Autodesk Inventor part; units mm, degrees
(part 2 of 9)
sketch "Sketch19" plane through (0, 0, 0) normal (1, 0, 0) x (0, 0, -1)
  arc A0 (177.0893, 15.8819) -> (169.6939, 53.0738) centre (0, 0) ccw projected
  line L0 (174.1799, 12.7) -> (91.821, 12.7) projected
  line L1 (88.9, 15.621) -> (88.9, 17.1891) projected
  line L2 (90.5865, 19.8364) -> (165.6716, 54.8492) projected
  line L3 (88.9, -0.254) -> (88.9, 0.254) projected
  line L4 (91.821, 3.175) -> (174.4218, 3.175) projected
  line L5 (177.3428, 0.254) -> (177.3428, -0.254) projected
  line L6 (174.4218, -3.175) -> (91.821, -3.175) projected
  line L7 (149.831, -89.2272) -> (89.9434, -38.9755) projected
  line L8 (88.9, -36.7379) -> (88.9, -15.621) projected
  line L9 (91.821, -12.7) -> (174.1799, -12.7) projected
  arc A1 (154.2425, -88.4425) -> (177.0893, -15.8819) centre (0, 0) ccw projected
  line L10 (-35.2916, -50.8) -> (42.0514, -50.8) projected
  arc A2 (74.705, -62.6849) -> (42.0514, -50.8) centre (42.0514, -101.6) ccw projected
  line L11 (74.705, -62.6849) -> (143.4787, -120.3929) projected
  arc A3 (143.8351, -124.9069) -> (143.4787, -120.3929) centre (141.4378, -122.8251) ccw projected
  arc A4 (141.8978, -127.1034) -> (143.8351, -124.9069) centre (0, 0) ccw projected
  arc A5 (141.8978, -127.1034) -> (141.494, -128.2246) centre (143.0803, -128.1626) ccw projected
  line L12 (141.6194, -131.4328) -> (141.494, -128.2246) projected
  arc A6 (141.6194, -131.4328) -> (142.123, -132.5318) centre (143.2057, -131.3708) ccw projected
  line L13 (142.123, -132.5318) -> (176.2311, -164.3381) projected
  arc A7 (176.2311, -164.3381) -> (194.6236, -163.2104) centre (184.8924, -155.0499) ccw projected
  arc A8 (194.6236, -163.2104) -> (235.5329, 95.0804) centre (0, 0) ccw projected
  arc A9 (235.5329, 95.0804) -> (218.389, 101.8364) centre (223.7562, 90.3263) ccw projected
  line L14 (218.389, 101.8364) -> (173.6183, 80.9596) projected
  arc A10 (152.1493, 76.2) -> (173.6183, 80.9596) centre (152.1493, 127) ccw projected
  line L15 (152.1493, 76.2) -> (-101.6, 76.2) projected
  line L16 (-101.6, 76.2) -> (-199.482, -21.682) projected
  line L17 (-199.482, -21.682) -> (-199.482, -255.599) projected
  line L18 (-199.482, -255.599) -> (-35.2916, -255.599) projected
  line L19 (-35.2916, -255.599) -> (-35.2916, -50.8) projected
  circle A11 centre (221.404, -95.9477) radius 3.3782 projected
  circle A12 centre (239.2356, 31.496) radius 3.3782 projected
  circle A13 centre (223.7295, 90.3926) radius 3.3782 projected
  circle A14 centre (239.2356, -31.496) radius 3.3782 projected
  arc A15 (180.8991, -105.7674) -> (203.0448, 51.8076) centre (0, 0) ccw projected
  line L20 (204.8485, 54.889) -> (206.0753, 55.2177) projected
  arc A16 (186.3731, -108.9857) -> (209.1938, 53.3924) centre (0, 0) ccw projected
  line L21 (182.8723, -109.8807) -> (181.7836, -109.2266) projected
  arc A17 (159.1231, -92.6879) -> (178.5072, 45.237) centre (0, 0) ccw projected
  line L22 (180.312, 48.3145) -> (181.5388, 48.6432) projected
  arc A18 (164.6013, -95.8992) -> (184.6584, 46.8139) centre (0, 0) ccw projected
  line L23 (161.0985, -96.7977) -> (160.0098, -96.1436) projected
  line L24 (171.9854, -103.3393) -> (170.8967, -102.6851) projected
  arc A19 (170.0112, -99.2275) -> (190.7761, 48.5222) centre (0, 0) ccw projected
  line L25 (192.5803, 51.6017) -> (193.8071, 51.9305) projected
  arc A20 (175.4872, -102.4426) -> (196.9261, 50.1033) centre (0, 0) ccw projected
  circle A21 centre (160.7915, -118.9794) radius 2.5527 projected
  circle A22 centre (0, 0) radius 13.335 projected
  line L26 (-110.3931, -99.2933) -> (-93.0185, -51.5569)
  line L27 (-101.8395, -100.8579) -> (-101.8395, -50.0579)
  line L28 (-110.6604, -51.6228) -> (-93.2858, -99.3592)
  line L29 (-118.4334, -56.0666) -> (-85.7798, -94.9817)
  line L30 (-124.2369, -62.8574) -> (-80.2428, -88.2574)
  arc A23 (88.9, -36.7379) -> (89.9434, -38.9755) centre (91.821, -36.7379) ccw projected
  arc A24 (91.821, -12.7) -> (88.9, -15.621) centre (91.821, -15.621) ccw projected
  arc A25 (177.0893, -15.8819) -> (174.1799, -12.7) centre (174.1799, -15.621) ccw projected
  arc A26 (149.831, -89.2272) -> (154.2425, -88.4425) centre (151.7086, -86.9895) ccw projected
  arc A27 (91.821, 3.175) -> (88.9, 0.254) centre (91.821, 0.254) ccw projected
  arc A28 (177.3428, 0.254) -> (174.4218, 3.175) centre (174.4218, 0.254) ccw projected
  arc A29 (174.4218, -3.175) -> (177.3428, -0.254) centre (174.4218, -0.254) ccw projected
  arc A30 (88.9, -0.254) -> (91.821, -3.175) centre (91.821, -0.254) ccw projected
  arc A31 (174.1799, 12.7) -> (177.0893, 15.8819) centre (174.1799, 15.621) ccw projected
  arc A32 (88.9, 15.621) -> (91.821, 12.7) centre (91.821, 15.621) ccw projected
  arc A33 (90.5865, 19.8364) -> (88.9, 17.1891) centre (91.821, 17.1891) ccw projected
  arc A34 (169.6939, 53.0738) -> (165.6716, 54.8492) centre (166.9061, 52.2019) ccw projected
  arc A35 (204.8485, 54.889) -> (203.0448, 51.8076) centre (205.5059, 52.4355) ccw projected
  arc A36 (209.1938, 53.3924) -> (206.0753, 55.2177) centre (206.7327, 52.7643) ccw projected
  arc A37 (182.8723, -109.8807) -> (186.3731, -108.9857) centre (184.1805, -107.7035) ccw projected
  arc A38 (180.8991, -105.7674) -> (181.7836, -109.2266) centre (183.0918, -107.0494) ccw projected
  arc A39 (180.312, 48.3145) -> (178.5072, 45.237) centre (180.9694, 45.861) ccw projected
  arc A40 (184.6584, 46.8139) -> (181.5388, 48.6432) centre (182.1962, 46.1897) ccw projected
  arc A41 (161.0985, -96.7977) -> (164.6013, -95.8992) centre (162.4067, -94.6205) ccw projected
  arc A42 (159.1231, -92.6879) -> (160.0098, -96.1436) centre (161.3179, -93.9664) ccw projected
  arc A43 (170.0112, -99.2275) -> (170.8967, -102.6851) centre (172.2049, -100.5079) ccw projected
  arc A44 (192.5803, 51.6017) -> (190.7761, 48.5222) centre (193.2377, 49.1483) ccw projected
  arc A45 (196.9261, 50.1033) -> (193.8071, 51.9305) centre (194.4645, 49.477) ccw projected
  arc A46 (171.9854, -103.3393) -> (175.4872, -102.4426) centre (173.2936, -101.1621) ccw projected
  arc A47 (-99.6119, -84.758) -> (-99.4903, -84.728) centre (-101.8395, -75.4579) ccw projected
  circle A48 centre (239.2356, -31.496) radius 3.3782 projected
  circle A49 centre (223.7295, 90.3926) radius 3.3782 projected
  circle A50 centre (239.2356, 31.496) radius 3.3782 projected
  circle A51 centre (221.404, -95.9477) radius 3.3782 projected
  line L31 (-35.2916, -50.8) -> (42.0514, -50.8) projected
  arc A52 (74.705, -62.6849) -> (42.0514, -50.8) centre (42.0514, -101.6) ccw projected
  line L32 (74.705, -62.6849) -> (143.4787, -120.3929) projected
  arc A53 (143.8351, -124.9069) -> (143.4787, -120.3929) centre (141.4378, -122.8251) ccw projected
  arc A54 (141.8978, -127.1034) -> (143.8351, -124.9069) centre (0, 0) ccw projected
  arc A55 (141.8978, -127.1034) -> (141.494, -128.2246) centre (143.0803, -128.1626) ccw projected
  line L33 (141.6194, -131.4328) -> (141.494, -128.2246) projected
  arc A56 (141.6194, -131.4328) -> (142.123, -132.5318) centre (143.2057, -131.3708) ccw projected
  line L34 (142.123, -132.5318) -> (176.2311, -164.3381) projected
  arc A57 (176.2311, -164.3381) -> (194.6236, -163.2104) centre (184.8924, -155.0499) ccw projected
  arc A58 (194.6236, -163.2104) -> (235.5329, 95.0804) centre (0, 0) ccw projected
  arc A59 (235.5329, 95.0804) -> (218.389, 101.8364) centre (223.7562, 90.3263) ccw projected
  line L35 (218.389, 101.8364) -> (173.6183, 80.9596) projected
  arc A60 (152.1493, 76.2) -> (173.6183, 80.9596) centre (152.1493, 127) ccw projected
  line L36 (152.1493, 76.2) -> (-101.6, 76.2) projected
  line L37 (-101.6, 76.2) -> (-199.482, -21.682) projected
  line L38 (-199.482, -21.682) -> (-199.482, -255.599) projected
  line L39 (-199.482, -255.599) -> (-35.2916, -255.599) projected
  line L40 (-35.2916, -255.599) -> (-35.2916, -50.8) projected
  line L41 (149.831, -89.2272) -> (89.9434, -38.9755) projected
  arc A61 (88.9, -36.7379) -> (89.9434, -38.9755) centre (91.821, -36.7379) ccw projected
  line L42 (88.9, -36.7379) -> (88.9, -15.621) projected
  arc A62 (91.821, -12.7) -> (88.9, -15.621) centre (91.821, -15.621) ccw projected
  line L43 (91.821, -12.7) -> (174.1799, -12.7) projected
  arc A63 (177.0893, -15.8819) -> (174.1799, -12.7) centre (174.1799, -15.621) ccw projected
  arc A64 (154.2425, -88.4425) -> (177.0893, -15.8819) centre (0, 0) ccw projected
  arc A65 (149.831, -89.2272) -> (154.2425, -88.4425) centre (151.7086, -86.9895) ccw projected
  line L44 (88.9, -0.254) -> (88.9, 0.254) projected
  arc A66 (91.821, 3.175) -> (88.9, 0.254) centre (91.821, 0.254) ccw projected
  line L45 (91.821, 3.175) -> (174.4218, 3.175) projected
  arc A67 (177.3428, 0.254) -> (174.4218, 3.175) centre (174.4218, 0.254) ccw projected
  line L46 (177.3428, 0.254) -> (177.3428, -0.254) projected
  arc A68 (174.4218, -3.175) -> (177.3428, -0.254) centre (174.4218, -0.254) ccw projected
  line L47 (174.4218, -3.175) -> (91.821, -3.175) projected
  arc A69 (88.9, -0.254) -> (91.821, -3.175) centre (91.821, -0.254) ccw projected
  arc A70 (177.0893, 15.8819) -> (169.6939, 53.0738) centre (0, 0) ccw projected
  arc A71 (174.1799, 12.7) -> (177.0893, 15.8819) centre (174.1799, 15.621) ccw projected
  line L48 (174.1799, 12.7) -> (91.821, 12.7) projected
  arc A72 (88.9, 15.621) -> (91.821, 12.7) centre (91.821, 15.621) ccw projected
  line L49 (88.9, 15.621) -> (88.9, 17.1891) projected
  arc A73 (90.5865, 19.8364) -> (88.9, 17.1891) centre (91.821, 17.1891) ccw projected
  line L50 (90.5865, 19.8364) -> (165.6716, 54.8492) projected
  arc A74 (169.6939, 53.0738) -> (165.6716, 54.8492) centre (166.9061, 52.2019) ccw projected
  arc A75 (180.8991, -105.7674) -> (203.0448, 51.8076) centre (0, 0) ccw projected
  arc A76 (204.8485, 54.889) -> (203.0448, 51.8076) centre (205.5059, 52.4355) ccw projected
  line L51 (204.8485, 54.889) -> (206.0753, 55.2177) projected
  arc A77 (209.1938, 53.3924) -> (206.0753, 55.2177) centre (206.7327, 52.7643) ccw projected
  arc A78 (186.3731, -108.9857) -> (209.1938, 53.3924) centre (0, 0) ccw projected
  arc A79 (182.8723, -109.8807) -> (186.3731, -108.9857) centre (184.1805, -107.7035) ccw projected
  line L52 (182.8723, -109.8807) -> (181.7836, -109.2266) projected
  arc A80 (180.8991, -105.7674) -> (181.7836, -109.2266) centre (183.0918, -107.0494) ccw projected
  arc A81 (159.1231, -92.6879) -> (178.5072, 45.237) centre (0, 0) ccw projected
  arc A82 (180.312, 48.3145) -> (178.5072, 45.237) centre (180.9694, 45.861) ccw projected
  line L53 (180.312, 48.3145) -> (181.5388, 48.6432) projected
  arc A83 (184.6584, 46.8139) -> (181.5388, 48.6432) centre (182.1962, 46.1897) ccw projected
  arc A84 (164.6013, -95.8992) -> (184.6584, 46.8139) centre (0, 0) ccw projected
  arc A85 (161.0985, -96.7977) -> (164.6013, -95.8992) centre (162.4067, -94.6205) ccw projected
  line L54 (161.0985, -96.7977) -> (160.0098, -96.1436) projected
  arc A86 (159.1231, -92.6879) -> (160.0098, -96.1436) centre (161.3179, -93.9664) ccw projected
  line L55 (171.9854, -103.3393) -> (170.8967, -102.6851) projected
  arc A87 (170.0112, -99.2275) -> (170.8967, -102.6851) centre (172.2049, -100.5079) ccw projected
  arc A88 (170.0112, -99.2275) -> (190.7761, 48.5222) centre (0, 0) ccw projected
  arc A89 (192.5803, 51.6017) -> (190.7761, 48.5222) centre (193.2377, 49.1483) ccw projected
  line L56 (192.5803, 51.6017) -> (193.8071, 51.9305) projected
  arc A90 (196.9261, 50.1033) -> (193.8071, 51.9305) centre (194.4645, 49.477) ccw projected
  arc A91 (175.4872, -102.4426) -> (196.9261, 50.1033) centre (0, 0) ccw projected
  arc A92 (171.9854, -103.3393) -> (175.4872, -102.4426) centre (173.2936, -101.1621) ccw projected
  circle A93 centre (187.962, 68.4126) radius 2.5527 projected
  circle A94 centre (160.7915, -118.9794) radius 2.5527 projected
  circle A95 centre (0, 0) radius 13.335 projected
  circle A96 centre (0, 0) radius 14.2875
  circle A97 centre (-101.8395, -75.4579) radius 31.75
  line L57 (-135.7109, 9.1855) -> (-95.7493, -10.2792)
  line L58 (-95.7493, -10.2792) -> (-76.2846, 29.6824)
  line L59 (-76.2846, 29.6824) -> (-116.2462, 49.1471)
  line L60 (-116.2462, 49.1471) -> (-135.7109, 9.1855)
  line L61 (-135.7109, 9.1855) -> (-76.2846, 29.6824) construction
  line L62 (-95.7493, -10.2792) -> (-116.2462, 49.1471) construction
  circle A98 centre (-101.8395, -75.4579) radius 44.565
  circle A99 centre (0, 0) radius 15.915
  line L63 (-119.5903, -34.5807) -> (-6.3391, 14.598)
  line L64 (-67.9013, -104.3411) -> (12.12, -10.3147)
  circle A100 centre (0, 0) radius 47.752
  line L65 (-107.8805, 35.2378) -> (-5.6488, 47.4167)
  circle A101 centre (-105.9978, 19.434) radius 15.9156
  line L66 (-113.3646, 5.3259) -> (-22.1029, -42.3286)
  line L67 (-100.3552, 14.7516) -> (-107.2315, 12.2061)
  line L68 (-107.2315, 12.2061) -> (-112.8741, 16.8885)
  line L69 (-112.8741, 16.8885) -> (-111.6404, 24.1163)
  line L70 (-111.6404, 24.1163) -> (-104.764, 26.6618)
  line L71 (-104.764, 26.6618) -> (-99.1214, 21.9794)
  line L72 (-99.1214, 21.9794) -> (-100.3552, 14.7516)
  circle A102 centre (-105.9978, 19.434) radius 7.3323
  circle A103 centre (-101.8395, -75.4579) radius 9.5631
  circle A104 centre (-105.9978, 19.434) radius 9.5631
  circle A105 centre (-101.8395, -75.4579) radius 25.4
  circle A106 centre (-105.9978, 19.434) radius 25.4
  line L73 (-101.8395, -75.4579) -> (0, 0)
  circle A107 centre (0, 0) radius 50.8
  circle A108 centre (-105.9978, 19.434) radius 31.4309
  arc A109 (136.2027, -114.2876) -> (161.1415, 75.1415) centre (0, 0) ccw
  line L74 (0, 0) -> (136.2027, -114.2876)
  line L75 (0, 0) -> (121.5323, 0)
  circle A110 centre (33.8645, -135.5333) radius 88.9
  circle A111 centre (-76.4174, -178.6042) radius 25.4
  line L76 (-88.4199, -21.0451) -> (-93.4785, -9.396)
  circle A112 centre (-76.4174, -178.6042) radius 21.4859
  line L77 (-141.7593, -95.2683) -> (-95.6637, -188.1553)
  line L78 (-57.286, -74.4485) -> (-54.9371, -178.1175)
  line L79 (136.2027, -114.2876) -> (98.8613, -216.8823)
  circle A113 centre (31.6927, -141.5004) radius 88.9
  line L80 (-52.5492, -187.2916) -> (90.6599, -239.4154)
  line L81 (-105.9978, 19.434) -> (0, 0)
  line L82 (-76.4174, -204.0042) -> (-76.4174, -178.6042)
  line L83 (136.2027, -114.2876) -> (136.2027, -216.8823)
  line L84 (-58.8554, 19.434) -> (-105.9978, 19.434)
  circle A114 centre (-17.4502, -276.5193) radius 88.9
  line L85 (-505.6291, -432.7823) -> (244.3318, -432.7823)
  circle A115 centre (-54.61, -343.8823) radius 88.9
  line L86 (-54.61, -258.1573) -> (-16.51, -258.1573)
  line L87 (-16.51, -258.1573) -> (-16.51, -340.7073)
  line L88 (-16.51, -340.7073) -> (-54.61, -340.7073)
  line L89 (-54.61, -340.7073) -> (-54.61, -258.1573)
  line L90 (-54.61, -299.4323) -> (-16.51, -299.4323)
  line L91 (-54.61, -343.8823) -> (-54.61, -254.9823)
  circle A116 centre (-16.51, -254.9823) radius 88.9
  line L92 (-16.51, -254.9823) -> (-16.51, -343.8823)
  circle A117 centre (-180.2765, -142.3655) radius 31.75
  circle A118 centre (-180.2765, -142.3655) radius 25.4
  circle A119 centre (-180.2765, -142.3655) radius 44.563
  circle A120 centre (-180.2765, -142.3655) radius 9.5631
  line L93 (-194.9575, -184.4408) -> (-91.0984, -220.6795)
  line L94 (-165.5955, -100.2902) -> (-61.7364, -136.5289)
  circle A121 centre (-76.4174, -178.6042) radius 44.563
  line L95 (-167.0299, -113.5109) -> (-119.1112, -9.1307)
  line L96 (-156.1209, -121.7605) -> (-135.7449, -104.3796)
  circle A122 centre (29.8359, -136.4768) radius 88.9
  line L97 (-116.4833, -117.4265) -> (-112.2994, -105.4355)
  circle A123 centre (-76.4174, -178.6042) radius 106.233
  arc A124 (-99.4903, -84.728) -> (-104.0551, -66.155) centre (-101.7058, -75.4251) ccw projected
  arc A125 (-99.7334, -84.7881) -> (-99.6119, -84.758) centre (-101.9731, -75.491) ccw projected
  arc A126 (-99.8547, -84.8183) -> (-99.7334, -84.7881) centre (-102.1066, -75.5241) ccw projected
  arc A127 (-104.4917, -66.2632) -> (-99.8547, -84.8183) centre (-102.2399, -75.5574) ccw projected
  arc A128 (-104.3463, -66.227) -> (-104.4917, -66.2632) centre (-102.1066, -75.5241) ccw projected
  arc A129 (-104.2008, -66.1909) -> (-104.3463, -66.227) centre (-101.9731, -75.491) ccw projected
  arc A130 (-104.0551, -66.155) -> (-104.2008, -66.1909) centre (-101.8395, -75.4579) ccw projected
  point P0 (-101.7058, -75.4251)
  point P1 (-101.9731, -75.491)
  point P2 (-102.1066, -75.5241)
  point P3 (-102.2399, -75.5574)
  point P4 (-35.56, -299.4323)
  dimension "d637" = 63.5
  dimension "d249" = 50.8
  dimension "d250" = 20
  dimension "d251" = 20
  dimension "d252" = 20
  dimension "d253" = 20
  dimension "d636" = 28.575
  dimension "d638" = 44.45
  dimension "d639" = 31.83
  dimension "d640" = 89.13
  dimension "d641" = 95.504
  dimension "d642" = 31.8313
  dimension "d643" = 12.7
  dimension "d644" = 19.1262
  dimension "d645" = 19.1262
  dimension "d646" = 50.8
  dimension "d647" = 50.8
  dimension "d648" = 107.7646
  dimension "d649" = 126.7485
  dimension "d650" = 101.6
  dimension "d651" = 127
  dimension "d652" = 40
  dimension "d653" = 177.8
  dimension "d654" = 50.8
  dimension "d655" = 12.7
  dimension "d656" = 6.35
  dimension "d657" = 106.233
  dimension "d658" = 152.4
  dimension "d659" = 279.1458
  dimension "d660" = 25
  dimension "d661" = 20
  dimension "d662" = 47.1424
  dimension "d663" = 42.9717
  dimension "d664" = 82.55
  dimension "d665" = 38.1
  dimension "d666" = 21.5575
  dimension "d667" = 35.56
  dimension "d668" = 215.9
  dimension "d669" = 215.9
  dimension "d670" = 26.7819
  dimension "d671" = 109.9998
  dimension "d672" = 432.7823
  dimension "d673" = 12.7
  dimension "d674" = 89.1261
  dimension "d675" = 126.6215
  dimension "d676" = 126.8755
  dimension "d677" = 127.0025
  dimension "d678" = 127.1295
  constraints: 92 end point, 31 point on circle, 28 coincident, 24 centre point, 24 tangent, 14 midpoint, 6 equal radius, 6 line through centre, 6 perpendicular, 6 point on line, 5 equal length, 5 horizontal, 5 vertical, 4 parallel, 3 concentric, 2 vertical alignment, 26 other
  measures "d249" distance of L26.start L26.end
  measures "d250" angle of L26 L27
  measures "d251" angle of L27 L28
  measures "d252" angle of L28 L29
  measures "d253" angle of L29 L30
  measures "d636" diameter of A96
  measures "d638" distance of L57.end L58.end
  measures "d639" diameter of A99
  measures "d640" diameter of A98
  measures "d641" diameter of A100
  measures "d642" diameter of A101
  measures "d643" distance between parallel lines of L71 L68
  measures "d644" diameter of A103
  measures "d645" diameter of A104
  measures "d646" diameter of A105
  measures "d647" diameter of A106
  measures "d648" distance of A96.centre point (-105.998, 19.434)
  measures "d649" distance of point (0, 0) point (-101.84, -75.458)
  measures "d650" diameter of A107
  measures "d651" radial gap between concentric circles of A109 A107
  measures "d652" angle of L75 L74
  measures "d653" diameter of A110
  measures "d654" diameter of A111
  measures "d655" distance of L76.start L76.end
  measures "d656" distance of A113.centre A110.centre
  measures "d657" distance of A123.start A111.centre
  measures "d658" distance of L80.start L80.end
  measures "d659" vertical distance of L82.start A109.end
  measures "d661" angle of L83 L79
  measures "d662" distance of point (-105.998, 19.434) L84.start
  measures "d663" diameter of A112
  measures "d664" distance of L88.end L86.start
  measures "d665" distance of L88.start L88.end
  measures "d666" distance of L92.start A114.centre
  measures "d667" horizontal distance of A107.centre point (-35.56, -299.432)
  measures "d668" distance from line of L85 L83.end
  measures "d669" distance from line of L85 L79.end
  measures "d670" distance of L96.start L96.end
  measures "d671" distance of A117.centre L82.end
  measures "d672" distance from line of L85 L74.start
  measures "d673" distance of L97.start L97.end
  measures "d674" diameter of A119
  measures "d675" distance of point (0, 0) A123.end
  measures "d676" distance of L73.end point (-101.973, -75.491)
  measures "d677" distance of L73.end point (-102.107, -75.524)
  measures "d678" distance of A58.centre point (-102.24, -75.557)
hole "Hole6" at (0, -51.6228, 110.6604) at (0, -99.3592, 93.2858) at (0, -62.8574, 124.2369) at (0, -56.0666, 118.4334) at (0, -50.0579, 101.8395) at (0, -51.5569, 93.0185) at (0, -99.2933, 110.3931) at (0, -100.8579, 101.8395) at (0, -94.9817, 85.7798) at (0, -88.2574, 80.2428) direction (-1, 0, 0) diameter 4.9784 end through all clearance for "Flat Head Machine Screw (82)" size "#10" standard "Ansi Unified Screw Threads"
sketch "Sketch22" plane through (0, 0, 0) normal (1, 0, 0) x (0, 0, -1)
  circle A0 centre (-85.7798, -94.9817) radius 2.4892 projected
  circle A1 centre (-110.3931, -99.2933) radius 2.4892 projected
  circle A2 centre (-101.8395, -50.0579) radius 2.4892 projected
  circle A3 centre (-124.2369, -62.8574) radius 2.4892 projected
  circle A4 centre (-110.6604, -51.6228) radius 2.4892 projected
  circle A5 centre (-93.2858, -99.3592) radius 2.4892 projected
  circle A6 centre (-118.4334, -56.0666) radius 2.4892 projected
  circle A7 centre (-93.0185, -51.5569) radius 2.4892 projected
  circle A8 centre (-101.8395, -100.8579) radius 2.4892 projected
  circle A9 centre (-80.2428, -88.2574) radius 2.4892 projected
  arc A10 (-99.4903, -84.728) -> (-104.0551, -66.155) centre (-101.7058, -75.4251) ccw projected
  arc A11 (-99.6119, -84.758) -> (-99.4903, -84.728) centre (-101.8395, -75.4579) ccw projected
  arc A12 (-99.7334, -84.7881) -> (-99.6119, -84.758) centre (-101.9731, -75.491) ccw projected
  arc A13 (-99.8547, -84.8183) -> (-99.7334, -84.7881) centre (-102.1066, -75.5241) ccw projected
  arc A14 (-104.4917, -66.2632) -> (-99.8547, -84.8183) centre (-102.2399, -75.5574) ccw projected
  arc A15 (-104.3463, -66.227) -> (-104.4917, -66.2632) centre (-102.1066, -75.5241) ccw projected
  arc A16 (-104.2008, -66.1909) -> (-104.3463, -66.227) centre (-101.9731, -75.491) ccw projected
  arc A17 (-104.0551, -66.155) -> (-104.2008, -66.1909) centre (-101.8395, -75.4579) ccw projected
  circle A18 centre (239.2356, -31.496) radius 3.3782 projected
  circle A19 centre (223.7295, 90.3926) radius 3.3782 projected
  circle A20 centre (239.2356, 31.496) radius 3.3782 projected
  circle A21 centre (221.404, -95.9477) radius 3.3782 projected
  line L0 (-35.2916, -50.8) -> (42.0514, -50.8) projected
  arc A22 (74.705, -62.6849) -> (42.0514, -50.8) centre (42.0514, -101.6) ccw projected
  line L1 (74.705, -62.6849) -> (143.4787, -120.3929) projected
  arc A23 (143.8351, -124.9069) -> (143.4787, -120.3929) centre (141.4378, -122.8251) ccw projected
  arc A24 (141.8978, -127.1034) -> (143.8351, -124.9069) centre (0, 0) ccw projected
  arc A25 (141.8978, -127.1034) -> (141.494, -128.2246) centre (143.0803, -128.1626) ccw projected
  line L2 (141.6194, -131.4328) -> (141.494, -128.2246) projected
  arc A26 (141.6194, -131.4328) -> (142.123, -132.5318) centre (143.2057, -131.3708) ccw projected
  line L3 (142.123, -132.5318) -> (176.2311, -164.3381) projected
  arc A27 (176.2311, -164.3381) -> (194.6236, -163.2104) centre (184.8924, -155.0499) ccw projected
  arc A28 (194.6236, -163.2104) -> (235.5329, 95.0804) centre (0, 0) ccw projected
  arc A29 (235.5329, 95.0804) -> (218.389, 101.8364) centre (223.7562, 90.3263) ccw projected
  line L4 (218.389, 101.8364) -> (173.6183, 80.9596) projected
  arc A30 (152.1493, 76.2) -> (173.6183, 80.9596) centre (152.1493, 127) ccw projected
  line L5 (152.1493, 76.2) -> (-101.6, 76.2) projected
  line L6 (-101.6, 76.2) -> (-199.482, -21.682) projected
  line L7 (-199.482, -21.682) -> (-199.482, -255.599) projected
  line L8 (-199.482, -255.599) -> (-35.2916, -255.599) projected
  line L9 (-35.2916, -255.599) -> (-35.2916, -50.8) projected
  line L10 (149.831, -89.2272) -> (89.9434, -38.9755) projected
  arc A31 (88.9, -36.7379) -> (89.9434, -38.9755) centre (91.821, -36.7379) ccw projected
  line L11 (88.9, -36.7379) -> (88.9, -15.621) projected
  arc A32 (91.821, -12.7) -> (88.9, -15.621) centre (91.821, -15.621) ccw projected
  line L12 (91.821, -12.7) -> (174.1799, -12.7) projected
  arc A33 (177.0893, -15.8819) -> (174.1799, -12.7) centre (174.1799, -15.621) ccw projected
  arc A34 (154.2425, -88.4425) -> (177.0893, -15.8819) centre (0, 0) ccw projected
  arc A35 (149.831, -89.2272) -> (154.2425, -88.4425) centre (151.7086, -86.9895) ccw projected
  line L13 (88.9, -0.254) -> (88.9, 0.254) projected
  arc A36 (91.821, 3.175) -> (88.9, 0.254) centre (91.821, 0.254) ccw projected
  line L14 (91.821, 3.175) -> (174.4218, 3.175) projected
  arc A37 (177.3428, 0.254) -> (174.4218, 3.175) centre (174.4218, 0.254) ccw projected
  line L15 (177.3428, 0.254) -> (177.3428, -0.254) projected
  arc A38 (174.4218, -3.175) -> (177.3428, -0.254) centre (174.4218, -0.254) ccw projected
  line L16 (174.4218, -3.175) -> (91.821, -3.175) projected
  arc A39 (88.9, -0.254) -> (91.821, -3.175) centre (91.821, -0.254) ccw projected
  arc A40 (177.0893, 15.8819) -> (169.6939, 53.0738) centre (0, 0) ccw projected
  arc A41 (174.1799, 12.7) -> (177.0893, 15.8819) centre (174.1799, 15.621) ccw projected
  line L17 (174.1799, 12.7) -> (91.821, 12.7) projected
  arc A42 (88.9, 15.621) -> (91.821, 12.7) centre (91.821, 15.621) ccw projected
  line L18 (88.9, 15.621) -> (88.9, 17.1891) projected
  arc A43 (90.5865, 19.8364) -> (88.9, 17.1891) centre (91.821, 17.1891) ccw projected
  line L19 (90.5865, 19.8364) -> (165.6716, 54.8492) projected
  arc A44 (169.6939, 53.0738) -> (165.6716, 54.8492) centre (166.9061, 52.2019) ccw projected
  arc A45 (180.8991, -105.7674) -> (203.0448, 51.8076) centre (0, 0) ccw projected
  arc A46 (204.8485, 54.889) -> (203.0448, 51.8076) centre (205.5059, 52.4355) ccw projected
  line L20 (204.8485, 54.889) -> (206.0753, 55.2177) projected
  arc A47 (209.1938, 53.3924) -> (206.0753, 55.2177) centre (206.7327, 52.7643) ccw projected
  arc A48 (186.3731, -108.9857) -> (209.1938, 53.3924) centre (0, 0) ccw projected
  arc A49 (182.8723, -109.8807) -> (186.3731, -108.9857) centre (184.1805, -107.7035) ccw projected
  line L21 (182.8723, -109.8807) -> (181.7836, -109.2266) projected
  arc A50 (180.8991, -105.7674) -> (181.7836, -109.2266) centre (183.0918, -107.0494) ccw projected
  arc A51 (159.1231, -92.6879) -> (178.5072, 45.237) centre (0, 0) ccw projected
  arc A52 (180.312, 48.3145) -> (178.5072, 45.237) centre (180.9694, 45.861) ccw projected
  line L22 (180.312, 48.3145) -> (181.5388, 48.6432) projected
  arc A53 (184.6584, 46.8139) -> (181.5388, 48.6432) centre (182.1962, 46.1897) ccw projected
  arc A54 (164.6013, -95.8992) -> (184.6584, 46.8139) centre (0, 0) ccw projected
  arc A55 (161.0985, -96.7977) -> (164.6013, -95.8992) centre (162.4067, -94.6205) ccw projected
  line L23 (161.0985, -96.7977) -> (160.0098, -96.1436) projected
  arc A56 (159.1231, -92.6879) -> (160.0098, -96.1436) centre (161.3179, -93.9664) ccw projected
  line L24 (171.9854, -103.3393) -> (170.8967, -102.6851) projected
  arc A57 (170.0112, -99.2275) -> (170.8967, -102.6851) centre (172.2049, -100.5079) ccw projected
  arc A58 (170.0112, -99.2275) -> (190.7761, 48.5222) centre (0, 0) ccw projected
  arc A59 (192.5803, 51.6017) -> (190.7761, 48.5222) centre (193.2377, 49.1483) ccw projected
  line L25 (192.5803, 51.6017) -> (193.8071, 51.9305) projected
  arc A60 (196.9261, 50.1033) -> (193.8071, 51.9305) centre (194.4645, 49.477) ccw projected
  arc A61 (175.4872, -102.4426) -> (196.9261, 50.1033) centre (0, 0) ccw projected
  arc A62 (171.9854, -103.3393) -> (175.4872, -102.4426) centre (173.2936, -101.1621) ccw projected
  circle A63 centre (187.962, 68.4126) radius 2.5527 projected
  circle A64 centre (160.7915, -118.9794) radius 2.5527 projected
  circle A65 centre (0, 0) radius 13.335 projected
  circle A66 centre (0, 0) radius 14.2875
  circle A67 centre (-101.8395, -75.4579) radius 31.75
  line L26 (-135.8009, 9.4503) -> (-96.0141, -10.3692)
  line L27 (-96.0141, -10.3692) -> (-76.1946, 29.4176)
  line L28 (-76.1946, 29.4176) -> (-115.9814, 49.2371)
  line L29 (-115.9814, 49.2371) -> (-135.8009, 9.4503)
  line L30 (-135.8009, 9.4503) -> (-76.1946, 29.4176) construction
  line L31 (-96.0141, -10.3692) -> (-115.9814, 49.2371) construction
  circle A68 centre (-101.8395, -75.4579) radius 44.565
  circle A69 centre (0, 0) radius 15.915
  line L32 (-119.5903, -34.5807) -> (-6.3391, 14.598)
  line L33 (-67.9013, -104.3411) -> (12.12, -10.3147)
  circle A70 centre (0, 0) radius 47.752
  line L34 (-107.8805, 35.2378) -> (-5.6488, 47.4167)
  circle A71 centre (-105.9978, 19.434) radius 15.9156
  line L35 (-113.3646, 5.3259) -> (-22.1029, -42.3286)
  line L36 (-100.3645, 14.7404) -> (-107.2459, 12.2086)
  line L37 (-107.2459, 12.2086) -> (-112.8792, 16.9022)
  line L38 (-112.8792, 16.9022) -> (-111.631, 24.1275)
  line L39 (-111.631, 24.1275) -> (-104.7496, 26.6593)
  line L40 (-104.7496, 26.6593) -> (-99.1164, 21.9657)
  line L41 (-99.1164, 21.9657) -> (-100.3645, 14.7404)
  circle A72 centre (-105.9978, 19.434) radius 7.3323
  circle A73 centre (-101.8395, -75.4579) radius 9.5631
  circle A74 centre (-105.9978, 19.434) radius 9.5631
  circle A75 centre (-101.8395, -75.4579) radius 25.4
  circle A76 centre (-105.9978, 19.434) radius 25.4
  line L42 (-101.8395, -75.4579) -> (0, 0)
  circle A77 centre (0, 0) radius 50.8
  circle A78 centre (-105.9978, 19.434) radius 31.4309
  arc A79 (136.2027, -114.2876) -> (161.1415, 75.1415) centre (0, 0) ccw
  line L43 (0, 0) -> (136.2027, -114.2876)
  line L44 (0, 0) -> (130.3807, 0)
  circle A80 centre (33.8645, -135.5333) radius 88.9
  circle A81 centre (-76.4174, -178.6042) radius 25.4
  line L45 (-88.4199, -21.0451) -> (-93.4785, -9.396)
  circle A82 centre (-76.4174, -178.6042) radius 21.4859
  line L46 (-141.7593, -95.2683) -> (-95.6637, -188.1553)
  line L47 (-57.286, -74.4485) -> (-54.9371, -178.1175)
  line L48 (136.2027, -114.2876) -> (90.5518, -239.7125)
  circle A83 centre (31.6927, -141.5004) radius 88.9
  line L49 (-52.5492, -187.2916) -> (90.6599, -239.4154)
  line L50 (-105.9978, 19.434) -> (0, 0)
  line L51 (-76.4174, -204.0042) -> (-76.4174, -178.6042)
  line L52 (136.2027, -114.2876) -> (136.2027, -239.7125)
  line L53 (-58.8554, 19.434) -> (-105.9978, 19.434)
  circle A84 centre (-17.4502, -276.5193) radius 88.9
  line L54 (-501.4434, -455.6125) -> (248.5176, -455.6125)
  line L55 (-550.7161, -581.025) -> (328.0098, -581.025)
  circle A85 centre (-54.61, -366.7125) radius 88.9
  line L56 (-54.61, -280.9875) -> (-16.51, -280.9875)
  line L57 (-16.51, -280.9875) -> (-16.51, -363.5375)
  line L58 (-16.51, -363.5375) -> (-54.61, -363.5375)
  line L59 (-54.61, -363.5375) -> (-54.61, -280.9875)
  line L60 (-54.61, -322.2625) -> (-16.51, -322.2625)
  line L61 (-54.61, -366.7125) -> (-54.61, -277.8125)
  circle A86 centre (-16.51, -277.8125) radius 88.9
  line L62 (-16.51, -277.8125) -> (-16.51, -366.7125)
  circle A87 centre (-180.2765, -142.3655) radius 31.75
  circle A88 centre (-180.2765, -142.3655) radius 25.4
  circle A89 centre (-180.2765, -142.3655) radius 44.563
  circle A90 centre (-180.2765, -142.3655) radius 9.5631
  line L63 (-194.9575, -184.4408) -> (-91.0984, -220.6795)
  line L64 (-165.5955, -100.2902) -> (-61.7364, -136.5289)
  circle A91 centre (-76.4174, -178.6042) radius 44.563
  line L65 (-167.0299, -113.5109) -> (-119.1112, -9.1307)
  line L66 (-156.1209, -121.7605) -> (-135.7449, -104.3796)
  circle A92 centre (29.8359, -136.4768) radius 88.9
  line L67 (-116.4833, -117.4265) -> (-112.2994, -105.4355)
  line L68 (-180.2765, -142.3655) -> (-76.4174, -178.6042)
  point P0 (-35.56, -322.2625)
  point P1 (-180.1566, -142.4074)
  point P2 (-180.3964, -142.3237)
  point P3 (-180.5163, -142.2818)
  point P4 (-180.3964, -142.3237)
  point P5 (-180.6362, -142.24)
  point P6 (-180.5163, -142.2818)
  dimension "d684" = 63.5
  dimension "d683" = 28.575
  dimension "d685" = 44.45
  dimension "d686" = 31.83
  dimension "d687" = 89.13
  dimension "d688" = 95.504
  dimension "d689" = 31.8313
  dimension "d690" = 12.7
  dimension "d691" = 19.1262
  dimension "d692" = 19.1262
  dimension "d693" = 50.8
  dimension "d694" = 50.8
  dimension "d695" = 107.7646
  dimension "d696" = 126.7485
  dimension "d697" = 101.6
  dimension "d698" = 127
  dimension "d699" = 40
  dimension "d700" = 177.8
  dimension "d701" = 50.8
  dimension "d702" = 12.7
  dimension "d703" = 6.35
  dimension "d704" = 106.233
  dimension "d705" = 152.4
  dimension "d706" = 279.1458
  dimension "d707" = 25
  dimension "d708" = 20
  dimension "d709" = 47.1424
  dimension "d710" = 42.9717
  dimension "d711" = 125.4125
  dimension "d712" = 656.1665
  dimension "d713" = 82.55
  dimension "d714" = 38.1
  dimension "d715" = 1.5989
  dimension "d716" = 35.56
  dimension "d717" = 215.9
  dimension "d718" = 215.9
  dimension "d719" = 26.7819
  dimension "d720" = 114.8539
  dimension "d721" = 109.9998
  dimension "d722" = 581.025
  dimension "d723" = 455.6125
  dimension "d724" = 12.7
  dimension "d725" = 89.1261
  dimension "d728" = 0.127
  dimension "d731" = 0.127
  constraints: 86 end point, 26 point on circle, 24 tangent, 23 centre point, 20 coincident, 9 midpoint, 7 perpendicular, 6 equal radius, 6 horizontal, 6 line through centre, 6 point on line, 4 parallel, 4 vertical, 3 concentric, 2 vertical alignment, 35 other
  measures "d683" diameter of A66
  measures "d685" distance of L27.start L27.end
  measures "d686" diameter of A69
  measures "d687" diameter of A68
  measures "d688" diameter of A70
  measures "d689" diameter of A71
  measures "d690" distance between parallel lines of L40 L37
  measures "d691" diameter of A73
  measures "d692" diameter of A74
  measures "d693" diameter of A75
  measures "d694" diameter of A76
  measures "d695" distance of A66.centre point (-105.998, 19.434)
  measures "d696" distance of point (0, 0) point (-101.84, -75.458)
  measures "d697" diameter of A77
  measures "d698" radial gap between concentric circles of A79 A77
  measures "d699" angle of L44 L43
  measures "d700" diameter of A80
  measures "d701" diameter of A81
  measures "d702" distance of L45.start L45.end
  measures "d703" distance of A83.centre A80.centre
  measures "d704" distance of point (-101.84, -75.458) A81.centre
  measures "d705" distance of L49.start L49.end
  measures "d706" vertical distance of L51.start A79.end
  measures "d708" angle of L52 L48
  measures "d709" distance of point (-105.998, 19.434) L53.start
  measures "d710" diameter of A82
  measures "d711" distance between parallel lines of L54 L55
  measures "d712" distance from line of A79.end L55
  measures "d713" distance of L58.end L59.end
  measures "d714" distance of L58.start L58.end
  measures "d715" distance of L62.start A84.centre
  measures "d716" horizontal distance of A77.centre point (-35.56, -322.262)
  measures "d717" distance from line of L54 L52.end
  measures "d718" distance from line of L54 L48.end
  measures "d719" distance of L66.start L66.end
  measures "d720" distance of L65.start L65.end
  measures "d721" distance of A87.centre L51.end
  measures "d722" distance from line of L55 point (0, 0)
  measures "d723" distance from line of L54 L43.start
  measures "d724" distance of L67.start L67.end
  measures "d725" diameter of A89
  measures "d728" distance of point (-180.277, -142.366) point (-180.157, -142.407)
  measures "d731" distance of point (-180.277, -142.366) point (-180.396, -142.324)
hole "Hole7" at (0, -142.24, 180.6362) at (0, -142.3237, 180.3964) at (0, -142.3655, 180.2765) at (0, -142.2818, 180.5163) at (0, -142.4074, 180.1566) direction (-1, 0, 0) diameter 19.1262 end through all
sketch "Sketch23" plane through (0, 0, 0) normal (1, 0, 0) x (0, 0, -1)
  circle A0 centre (0, 0) radius 13.335 projected
  circle A1 centre (160.7915, -118.9794) radius 2.5527 projected
  line L0 (182.8723, -109.8807) -> (181.7836, -109.2266) projected
  arc A2 (170.0112, -99.2275) -> (190.7761, 48.5222) centre (0, 0) ccw projected
  line L1 (204.8485, 54.889) -> (206.0753, 55.2177) projected
  arc A3 (175.4872, -102.4426) -> (196.9261, 50.1033) centre (0, 0) ccw projected
  arc A4 (159.1231, -92.6879) -> (178.5072, 45.237) centre (0, 0) ccw projected
  line L2 (180.312, 48.3145) -> (181.5388, 48.6432) projected
  arc A5 (164.6013, -95.8992) -> (184.6584, 46.8139) centre (0, 0) ccw projected
  line L3 (161.0985, -96.7977) -> (160.0098, -96.1436) projected
  arc A6 (180.8991, -105.7674) -> (203.0448, 51.8076) centre (0, 0) ccw projected
  line L4 (192.5803, 51.6017) -> (193.8071, 51.9305) projected
  arc A7 (186.3731, -108.9857) -> (209.1938, 53.3924) centre (0, 0) ccw projected
  line L5 (171.9854, -103.3393) -> (170.8967, -102.6851) projected
  circle A8 centre (239.2356, -31.496) radius 3.3782 projected
  circle A9 centre (223.7295, 90.3926) radius 3.3782 projected
  circle A10 centre (239.2356, 31.496) radius 3.3782 projected
  circle A11 centre (221.404, -95.9477) radius 3.3782 projected
  line L6 (-35.2916, -50.8) -> (42.0514, -50.8) projected
  arc A12 (74.705, -62.6849) -> (42.0514, -50.8) centre (42.0514, -101.6) ccw projected
  line L7 (74.705, -62.6849) -> (143.4787, -120.3929) projected
  arc A13 (143.8351, -124.9069) -> (143.4787, -120.3929) centre (141.4378, -122.8251) ccw projected
  arc A14 (141.8978, -127.1034) -> (143.8351, -124.9069) centre (0, 0) ccw projected
  arc A15 (141.8978, -127.1034) -> (141.494, -128.2246) centre (143.0803, -128.1626) ccw projected
  line L8 (141.6194, -131.4328) -> (141.494, -128.2246) projected
  arc A16 (141.6194, -131.4328) -> (142.123, -132.5318) centre (143.2057, -131.3708) ccw projected
  line L9 (142.123, -132.5318) -> (176.2311, -164.3381) projected
  arc A17 (176.2311, -164.3381) -> (194.6236, -163.2104) centre (184.8924, -155.0499) ccw projected
  arc A18 (194.6236, -163.2104) -> (235.5329, 95.0804) centre (0, 0) ccw projected
  arc A19 (235.5329, 95.0804) -> (218.389, 101.8364) centre (223.7562, 90.3263) ccw projected
  line L10 (218.389, 101.8364) -> (173.6183, 80.9596) projected
  arc A20 (152.1493, 76.2) -> (173.6183, 80.9596) centre (152.1493, 127) ccw projected
  line L11 (152.1493, 76.2) -> (-101.6, 76.2) projected
  line L12 (-101.6, 76.2) -> (-199.482, -21.682) projected
  line L13 (-199.482, -21.682) -> (-199.482, -255.599) projected
  line L14 (-199.482, -255.599) -> (-35.2916, -255.599) projected
  line L15 (-35.2916, -255.599) -> (-35.2916, -50.8) projected
  line L16 (149.831, -89.2272) -> (89.9434, -38.9755) projected
  line L17 (88.9, -36.7379) -> (88.9, -15.621) projected
  line L18 (91.821, -12.7) -> (174.1799, -12.7) projected
  arc A21 (154.2425, -88.4425) -> (177.0893, -15.8819) centre (0, 0) ccw projected
  line L19 (88.9, -0.254) -> (88.9, 0.254) projected
  line L20 (91.821, 3.175) -> (174.4218, 3.175) projected
  line L21 (177.3428, 0.254) -> (177.3428, -0.254) projected
  line L22 (174.4218, -3.175) -> (91.821, -3.175) projected
  arc A22 (177.0893, 15.8819) -> (169.6939, 53.0738) centre (0, 0) ccw projected
  line L23 (174.1799, 12.7) -> (91.821, 12.7) projected
  line L24 (88.9, 15.621) -> (88.9, 17.1891) projected
  line L25 (90.5865, 19.8364) -> (165.6716, 54.8492) projected
  circle A23 centre (-80.2428, -88.2574) radius 2.4892 projected
  circle A24 centre (-101.8395, -100.8579) radius 2.4892 projected
  circle A25 centre (-93.0185, -51.5569) radius 2.4892 projected
  circle A26 centre (-93.2858, -99.3592) radius 2.4892 projected
  circle A27 centre (-110.6604, -51.6228) radius 2.4892 projected
  circle A28 centre (-124.2369, -62.8574) radius 2.4892 projected
  circle A29 centre (-101.8395, -50.0579) radius 2.4892 projected
  circle A30 centre (-110.3931, -99.2933) radius 2.4892 projected
  circle A31 centre (-85.7798, -94.9817) radius 2.4892 projected
  line L26 (-187.1176, -166.8269) -> (-173.4354, -117.9041)
  line L27 (-168.1768, -164.3742) -> (-193.0957, -120.1058)
  line L28 (-180.6733, -167.7222) -> (-180.1195, -116.9252)
  line L29 (-174.2102, -166.8866) -> (-186.8225, -117.6771)
  line L30 (-193.0957, -164.2646) -> (-167.2175, -120.5501)
  arc A32 (174.1799, 12.7) -> (177.0893, 15.8819) centre (174.1799, 15.621) ccw projected
  arc A33 (88.9, 15.621) -> (91.821, 12.7) centre (91.821, 15.621) ccw projected
  arc A34 (90.5865, 19.8364) -> (88.9, 17.1891) centre (91.821, 17.1891) ccw projected
  arc A35 (169.6939, 53.0738) -> (165.6716, 54.8492) centre (166.9061, 52.2019) ccw projected
  arc A36 (91.821, 3.175) -> (88.9, 0.254) centre (91.821, 0.254) ccw projected
  arc A37 (177.3428, 0.254) -> (174.4218, 3.175) centre (174.4218, 0.254) ccw projected
  arc A38 (174.4218, -3.175) -> (177.3428, -0.254) centre (174.4218, -0.254) ccw projected
  arc A39 (88.9, -0.254) -> (91.821, -3.175) centre (91.821, -0.254) ccw projected
  arc A40 (88.9, -36.7379) -> (89.9434, -38.9755) centre (91.821, -36.7379) ccw projected
  arc A41 (91.821, -12.7) -> (88.9, -15.621) centre (91.821, -15.621) ccw projected
  arc A42 (177.0893, -15.8819) -> (174.1799, -12.7) centre (174.1799, -15.621) ccw projected
  arc A43 (149.831, -89.2272) -> (154.2425, -88.4425) centre (151.7086, -86.9895) ccw projected
  arc A44 (170.0112, -99.2275) -> (170.8967, -102.6851) centre (172.2049, -100.5079) ccw projected
  arc A45 (192.5803, 51.6017) -> (190.7761, 48.5222) centre (193.2377, 49.1483) ccw projected
  arc A46 (196.9261, 50.1033) -> (193.8071, 51.9305) centre (194.4645, 49.477) ccw projected
  arc A47 (171.9854, -103.3393) -> (175.4872, -102.4426) centre (173.2936, -101.1621) ccw projected
  arc A48 (180.312, 48.3145) -> (178.5072, 45.237) centre (180.9694, 45.861) ccw projected
  arc A49 (184.6584, 46.8139) -> (181.5388, 48.6432) centre (182.1962, 46.1897) ccw projected
  arc A50 (161.0985, -96.7977) -> (164.6013, -95.8992) centre (162.4067, -94.6205) ccw projected
  arc A51 (159.1231, -92.6879) -> (160.0098, -96.1436) centre (161.3179, -93.9664) ccw projected
  arc A52 (204.8485, 54.889) -> (203.0448, 51.8076) centre (205.5059, 52.4355) ccw projected
  arc A53 (209.1938, 53.3924) -> (206.0753, 55.2177) centre (206.7327, 52.7643) ccw projected
  arc A54 (182.8723, -109.8807) -> (186.3731, -108.9857) centre (184.1805, -107.7035) ccw projected
  arc A55 (180.8991, -105.7674) -> (181.7836, -109.2266) centre (183.0918, -107.0494) ccw projected
  arc A56 (-99.6119, -84.758) -> (-99.4903, -84.728) centre (-101.8395, -75.4579) ccw projected
  arc A57 (-99.4903, -84.728) -> (-104.0551, -66.155) centre (-101.7058, -75.4251) ccw projected
  arc A58 (-99.7334, -84.7881) -> (-99.6119, -84.758) centre (-101.9731, -75.491) ccw projected
  arc A59 (-99.8547, -84.8183) -> (-99.7334, -84.7881) centre (-102.1066, -75.5241) ccw projected
  arc A60 (-104.4917, -66.2632) -> (-99.8547, -84.8183) centre (-102.2399, -75.5574) ccw projected
  arc A61 (-104.3463, -66.227) -> (-104.4917, -66.2632) centre (-102.1066, -75.5241) ccw projected
  arc A62 (-104.2008, -66.1909) -> (-104.3463, -66.227) centre (-101.9731, -75.491) ccw projected
  arc A63 (-104.0551, -66.155) -> (-104.2008, -66.1909) centre (-101.8395, -75.4579) ccw projected
  arc A64 (-183.7267, -151.29) -> (-183.6068, -151.3318) centre (-180.5163, -142.2818) ccw projected
  arc A65 (-177.4258, -133.2319) -> (-183.7267, -151.29) centre (-180.6362, -142.24) ccw projected
  arc A66 (-177.3059, -133.2737) -> (-177.4258, -133.2319) centre (-180.5163, -142.2818) ccw projected
  arc A67 (-177.186, -133.3155) -> (-177.3059, -133.2737) centre (-180.3964, -142.3237) ccw projected
  arc A68 (-177.0661, -133.3574) -> (-177.186, -133.3155) centre (-180.2765, -142.3655) ccw projected
  arc A69 (-183.367, -151.4155) -> (-177.0661, -133.3574) centre (-180.1566, -142.4074) ccw projected
  arc A70 (-183.4869, -151.3736) -> (-183.367, -151.4155) centre (-180.2765, -142.3655) ccw projected
  arc A71 (-183.6068, -151.3318) -> (-183.4869, -151.3736) centre (-180.3964, -142.3237) ccw projected
  circle A72 centre (-85.7798, -94.9817) radius 2.4892 projected
  circle A73 centre (-110.3931, -99.2933) radius 2.4892 projected
  circle A74 centre (-101.8395, -50.0579) radius 2.4892 projected
  circle A75 centre (-124.2369, -62.8574) radius 2.4892 projected
  circle A76 centre (-110.6604, -51.6228) radius 2.4892 projected
  circle A77 centre (-93.2858, -99.3592) radius 2.4892 projected
  circle A78 centre (-118.4334, -56.0666) radius 2.4892 projected
  circle A79 centre (-93.0185, -51.5569) radius 2.4892 projected
  circle A80 centre (-101.8395, -100.8579) radius 2.4892 projected
  circle A81 centre (-80.2428, -88.2574) radius 2.4892 projected
  arc A82 (-99.4903, -84.728) -> (-104.0551, -66.155) centre (-101.7058, -75.4251) ccw projected
  arc A83 (-99.6119, -84.758) -> (-99.4903, -84.728) centre (-101.8395, -75.4579) ccw projected
  arc A84 (-99.7334, -84.7881) -> (-99.6119, -84.758) centre (-101.9731, -75.491) ccw projected
  arc A85 (-99.8547, -84.8183) -> (-99.7334, -84.7881) centre (-102.1066, -75.5241) ccw projected
  arc A86 (-104.4917, -66.2632) -> (-99.8547, -84.8183) centre (-102.2399, -75.5574) ccw projected
  arc A87 (-104.3463, -66.227) -> (-104.4917, -66.2632) centre (-102.1066, -75.5241) ccw projected
  arc A88 (-104.2008, -66.1909) -> (-104.3463, -66.227) centre (-101.9731, -75.491) ccw projected
  arc A89 (-104.0551, -66.155) -> (-104.2008, -66.1909) centre (-101.8395, -75.4579) ccw projected
  circle A90 centre (239.2356, -31.496) radius 3.3782 projected
  circle A91 centre (223.7295, 90.3926) radius 3.3782 projected
  circle A92 centre (239.2356, 31.496) radius 3.3782 projected
  circle A93 centre (221.404, -95.9477) radius 3.3782 projected
  line L31 (-35.2916, -50.8) -> (42.0514, -50.8) projected
  arc A94 (74.705, -62.6849) -> (42.0514, -50.8) centre (42.0514, -101.6) ccw projected
  line L32 (74.705, -62.6849) -> (143.4787, -120.3929) projected
  arc A95 (143.8351, -124.9069) -> (143.4787, -120.3929) centre (141.4378, -122.8251) ccw projected
  arc A96 (141.8978, -127.1034) -> (143.8351, -124.9069) centre (0, 0) ccw projected
  arc A97 (141.8978, -127.1034) -> (141.494, -128.2246) centre (143.0803, -128.1626) ccw projected
  line L33 (141.6194, -131.4328) -> (141.494, -128.2246) projected
  arc A98 (141.6194, -131.4328) -> (142.123, -132.5318) centre (143.2057, -131.3708) ccw projected
  line L34 (142.123, -132.5318) -> (176.2311, -164.3381) projected
  arc A99 (176.2311, -164.3381) -> (194.6236, -163.2104) centre (184.8924, -155.0499) ccw projected
  arc A100 (194.6236, -163.2104) -> (235.5329, 95.0804) centre (0, 0) ccw projected
  arc A101 (235.5329, 95.0804) -> (218.389, 101.8364) centre (223.7562, 90.3263) ccw projected
  line L35 (218.389, 101.8364) -> (173.6183, 80.9596) projected
  arc A102 (152.1493, 76.2) -> (173.6183, 80.9596) centre (152.1493, 127) ccw projected
  line L36 (152.1493, 76.2) -> (-101.6, 76.2) projected
  line L37 (-101.6, 76.2) -> (-199.482, -21.682) projected
  line L38 (-199.482, -21.682) -> (-199.482, -255.599) projected
  line L39 (-199.482, -255.599) -> (-35.2916, -255.599) projected
  line L40 (-35.2916, -255.599) -> (-35.2916, -50.8) projected
  line L41 (149.831, -89.2272) -> (89.9434, -38.9755) projected
  arc A103 (88.9, -36.7379) -> (89.9434, -38.9755) centre (91.821, -36.7379) ccw projected
  line L42 (88.9, -36.7379) -> (88.9, -15.621) projected
  arc A104 (91.821, -12.7) -> (88.9, -15.621) centre (91.821, -15.621) ccw projected
  line L43 (91.821, -12.7) -> (174.1799, -12.7) projected
  arc A105 (177.0893, -15.8819) -> (174.1799, -12.7) centre (174.1799, -15.621) ccw projected
  arc A106 (154.2425, -88.4425) -> (177.0893, -15.8819) centre (0, 0) ccw projected
  arc A107 (149.831, -89.2272) -> (154.2425, -88.4425) centre (151.7086, -86.9895) ccw projected
  line L44 (88.9, -0.254) -> (88.9, 0.254) projected
  arc A108 (91.821, 3.175) -> (88.9, 0.254) centre (91.821, 0.254) ccw projected
  line L45 (91.821, 3.175) -> (174.4218, 3.175) projected
  arc A109 (177.3428, 0.254) -> (174.4218, 3.175) centre (174.4218, 0.254) ccw projected
  line L46 (177.3428, 0.254) -> (177.3428, -0.254) projected
  arc A110 (174.4218, -3.175) -> (177.3428, -0.254) centre (174.4218, -0.254) ccw projected
  line L47 (174.4218, -3.175) -> (91.821, -3.175) projected
  arc A111 (88.9, -0.254) -> (91.821, -3.175) centre (91.821, -0.254) ccw projected
  arc A112 (177.0893, 15.8819) -> (169.6939, 53.0738) centre (0, 0) ccw projected
  arc A113 (174.1799, 12.7) -> (177.0893, 15.8819) centre (174.1799, 15.621) ccw projected
  line L48 (174.1799, 12.7) -> (91.821, 12.7) projected
  arc A114 (88.9, 15.621) -> (91.821, 12.7) centre (91.821, 15.621) ccw projected
  line L49 (88.9, 15.621) -> (88.9, 17.1891) projected
  arc A115 (90.5865, 19.8364) -> (88.9, 17.1891) centre (91.821, 17.1891) ccw projected
  line L50 (90.5865, 19.8364) -> (165.6716, 54.8492) projected
  arc A116 (169.6939, 53.0738) -> (165.6716, 54.8492) centre (166.9061, 52.2019) ccw projected
  arc A117 (180.8991, -105.7674) -> (203.0448, 51.8076) centre (0, 0) ccw projected
  arc A118 (204.8485, 54.889) -> (203.0448, 51.8076) centre (205.5059, 52.4355) ccw projected
  line L51 (204.8485, 54.889) -> (206.0753, 55.2177) projected
  arc A119 (209.1938, 53.3924) -> (206.0753, 55.2177) centre (206.7327, 52.7643) ccw projected
  arc A120 (186.3731, -108.9857) -> (209.1938, 53.3924) centre (0, 0) ccw projected
  arc A121 (182.8723, -109.8807) -> (186.3731, -108.9857) centre (184.1805, -107.7035) ccw projected
  line L52 (182.8723, -109.8807) -> (181.7836, -109.2266) projected
  arc A122 (180.8991, -105.7674) -> (181.7836, -109.2266) centre (183.0918, -107.0494) ccw projected
  arc A123 (159.1231, -92.6879) -> (178.5072, 45.237) centre (0, 0) ccw projected
  arc A124 (180.312, 48.3145) -> (178.5072, 45.237) centre (180.9694, 45.861) ccw projected
  line L53 (180.312, 48.3145) -> (181.5388, 48.6432) projected
  arc A125 (184.6584, 46.8139) -> (181.5388, 48.6432) centre (182.1962, 46.1897) ccw projected
  arc A126 (164.6013, -95.8992) -> (184.6584, 46.8139) centre (0, 0) ccw projected
  arc A127 (161.0985, -96.7977) -> (164.6013, -95.8992) centre (162.4067, -94.6205) ccw projected
  line L54 (161.0985, -96.7977) -> (160.0098, -96.1436) projected
  arc A128 (159.1231, -92.6879) -> (160.0098, -96.1436) centre (161.3179, -93.9664) ccw projected
  line L55 (171.9854, -103.3393) -> (170.8967, -102.6851) projected
  arc A129 (170.0112, -99.2275) -> (170.8967, -102.6851) centre (172.2049, -100.5079) ccw projected
  arc A130 (170.0112, -99.2275) -> (190.7761, 48.5222) centre (0, 0) ccw projected
  arc A131 (192.5803, 51.6017) -> (190.7761, 48.5222) centre (193.2377, 49.1483) ccw projected
  line L56 (192.5803, 51.6017) -> (193.8071, 51.9305) projected
  arc A132 (196.9261, 50.1033) -> (193.8071, 51.9305) centre (194.4645, 49.477) ccw projected
  arc A133 (175.4872, -102.4426) -> (196.9261, 50.1033) centre (0, 0) ccw projected
  arc A134 (171.9854, -103.3393) -> (175.4872, -102.4426) centre (173.2936, -101.1621) ccw projected
  circle A135 centre (187.962, 68.4126) radius 2.5527 projected
  circle A136 centre (160.7915, -118.9794) radius 2.5527 projected
  circle A137 centre (0, 0) radius 13.335 projected
  line L57 (-193.0957, -120.1058) -> (-199.482, -120.1058)
  line L58 (-199.482, -21.682) -> (-199.482, -255.599) projected
  line L59 (-193.0957, -164.2646) -> (-199.482, -164.2646)
  point P0 (-180.1566, -142.4074)
  point P1 (-180.3964, -142.3237)
  dimension "d321" = 50.8
  dimension "d322" = 15
  dimension "d323" = 15
  dimension "d324" = 15
  dimension "d325" = 15
  constraints: 15 coincident, 14 end point, 5 equal length, 5 midpoint, 2 point on line, 1 horizontal, 1 perpendicular
  measures "d321" distance of L26.start L26.end
  measures "d322" angle of L30 L26
  measures "d323" angle of L26 L28
  measures "d324" angle of L28 L29
  measures "d325" angle of L29 L27
hole "Hole8" at (0, -120.1058, 193.0957) at (0, -117.6771, 186.8225) at (0, -116.9252, 180.1195) at (0, -117.9041, 173.4354) at (0, -120.5501, 167.2175) at (0, -164.3742, 168.1768) at (0, -166.8866, 174.2102) at (0, -167.7222, 180.6733) at (0, -166.8269, 187.1176) at (0, -164.2646, 193.0957) direction (-1, 0, 0) diameter 4.9784 end through all clearance for "Flat Head Machine Screw (82)" size "#10" standard "Ansi Unified Screw Threads"